Autodesk Inventor part; units mm, degrees
(part 2 of 3)
  spline S197 degree 2 poles (-17.3831, 5.9159) (-17.3831, 6.0168) (-17.518, 6.1517) (-17.6383, 6.1517) knots 0 0 0 1 2 2 2
  spline S198 degree 2 poles (-17.6383, 6.1517) (-17.7477, 6.1517) (-17.8875, 6.0314) (-17.8875, 5.928) knots 0 0 0 1 2 2 2
  spline S199 degree 2 poles (-17.8875, 5.928) (-17.8875, 5.8539) (-17.8158, 5.7506) (-17.7441, 5.7092) knots 0 0 0 1 2 2 2
  spline S200 degree 2 poles (-17.7441, 5.7092) (-17.7137, 5.6922) (-17.5848, 5.6327) (-17.5326, 5.6156) knots 0 0 0 1 2 2 2
  spline S201 degree 2 poles (-17.5326, 5.6156) (-17.4451, 5.6825) (-17.3831, 5.8247) (-17.3831, 5.9159) knots 0 0 0 1 2 2 2
  line L310 (-16.9748, 4.9432) -> (-16.6479, 4.9432)
  spline S202 degree 2 poles (-16.6479, 4.9432) (-16.9588, 5.2027) (-16.9588, 5.5777) knots 0 0 0 1 1 1
  spline S203 degree 2 poles (-16.9588, 5.5777) (-16.9588, 5.7812) (-16.7953, 6.1048) (-16.4958, 6.2923) (-16.2866, 6.2923) knots 0 0 0 1 2 3 3 3
  spline S204 degree 2 poles (-16.2866, 6.2923) (-16.0785, 6.2923) (-15.8018, 6.1208) (-15.6223, 5.7984) (-15.6223, 5.5777) knots 0 0 0 1 2 3 3 3
  spline S205 degree 2 poles (-15.6223, 5.5777) (-15.6223, 5.2027) (-15.9322, 4.9432) knots 0 0 0 1 1 1
  line L311 (-15.9322, 4.9432) -> (-15.6063, 4.9432)
  line L312 (-15.6063, 4.9432) -> (-15.6063, 4.766)
  line L313 (-15.6063, 4.766) -> (-16.1883, 4.766)
  line L314 (-16.1883, 4.766) -> (-16.1883, 4.9317)
  spline S206 degree 2 poles (-16.1883, 4.9317) (-15.8247, 5.1021) (-15.8247, 5.5468) knots 0 0 0 1 1 1
  spline S207 degree 2 poles (-15.8247, 5.5468) (-15.8247, 5.7972) (-16.0819, 6.1219) (-16.2877, 6.1219) knots 0 0 0 1 2 2 2
  spline S208 degree 2 poles (-16.2877, 6.1219) (-16.5004, 6.1219) (-16.7542, 5.7949) (-16.7542, 5.5571) knots 0 0 0 1 2 2 2
  spline S209 degree 2 poles (-16.7542, 5.5571) (-16.7542, 5.1055) (-16.3906, 4.9317) knots 0 0 0 1 1 1
  line L315 (-16.3906, 4.9317) -> (-16.3906, 4.766)
  line L316 (-16.3906, 4.766) -> (-16.9748, 4.766)
  line L317 (-16.9748, 4.766) -> (-16.9748, 4.9432)
  line L318 (-14.3756, 5.0335) -> (-14.3756, 5.4451)
  line L319 (-14.3756, 5.4451) -> (-14.7837, 5.4451)
  line L320 (-14.7837, 5.4451) -> (-14.7837, 5.6154)
  line L321 (-14.7837, 5.6154) -> (-14.3756, 5.6154)
  line L322 (-14.3756, 5.6154) -> (-14.3756, 6.0236)
  line L323 (-14.3756, 6.0236) -> (-14.2018, 6.0236)
  line L324 (-14.2018, 6.0236) -> (-14.2018, 5.6154)
  line L325 (-14.2018, 5.6154) -> (-13.7936, 5.6154)
  line L326 (-13.7936, 5.6154) -> (-13.7936, 5.4451)
  line L327 (-13.7936, 5.4451) -> (-14.2018, 5.4451)
  line L328 (-14.2018, 5.4451) -> (-14.2018, 5.0335)
  line L329 (-14.2018, 5.0335) -> (-14.3756, 5.0335)
  line L330 (-13.7936, 4.766) -> (-14.7837, 4.766)
  line L331 (-14.7837, 4.766) -> (-14.7837, 4.9375)
  line L332 (-14.7837, 4.9375) -> (-13.7936, 4.9375)
  line L333 (-13.7936, 4.9375) -> (-13.7936, 4.766)
  line L334 (-12.1726, 4.766) -> (-12.9044, 4.766)
  line L335 (-12.9044, 4.766) -> (-12.9044, 4.9191)
  line L336 (-12.9044, 4.9191) -> (-12.6321, 4.9191)
  line L337 (-12.6321, 4.9191) -> (-12.6321, 5.9244)
  line L338 (-12.6321, 5.9244) -> (-12.9044, 5.9244)
  line L339 (-12.9044, 5.9244) -> (-12.9044, 6.0618)
  spline S210 degree 2 poles (-12.9044, 6.0618) (-12.75, 6.0618) (-12.6041, 6.1493) (-12.5944, 6.2708) knots 0 0 0 1 2 2 2
  line L340 (-12.5944, 6.2708) -> (-12.4388, 6.2708)
  line L341 (-12.4388, 6.2708) -> (-12.4388, 4.9191)
  line L342 (-12.4388, 4.9191) -> (-12.1726, 4.9191)
  line L343 (-12.1726, 4.9191) -> (-12.1726, 4.766)
  spline S211 degree 2 poles (-10.9631, 5.516) (-10.9631, 5.1124) (-11.1977, 4.7344) (-11.442, 4.7344) knots 0 0 0 1 2 2 2
  spline S212 degree 2 poles (-11.442, 4.7344) (-11.69, 4.7344) (-11.9222, 5.1197) (-11.9222, 5.5147) knots 0 0 0 1 2 2 2
  spline S213 degree 2 poles (-11.9222, 5.5147) (-11.9222, 5.9207) (-11.6876, 6.2964) (-11.442, 6.2964) knots 0 0 0 1 2 2 2
  spline S214 degree 2 poles (-11.442, 6.2964) (-11.1953, 6.2964) (-10.9631, 5.9074) (-10.9631, 5.516) knots 0 0 0 1 2 2 2
  spline S215 degree 2 poles (-11.2208, 5.0589) (-11.1916, 5.1331) (-11.1673, 5.3616) (-11.1673, 5.516) knots 0 0 0 1 2 2 2
  spline S216 degree 2 poles (-11.1673, 5.516) (-11.1673, 5.6703) (-11.1916, 5.8976) (-11.222, 5.9742) knots 0 0 0 1 2 2 2
  spline S217 degree 2 poles (-11.222, 5.9742) (-11.2524, 6.0508) (-11.3582, 6.1298) (-11.442, 6.1298) knots 0 0 0 1 2 2 2
  spline S218 degree 2 poles (-11.442, 6.1298) (-11.5259, 6.1298) (-11.6341, 6.0508) (-11.6657, 5.9718) knots 0 0 0 1 2 2 2
  spline S219 degree 2 poles (-11.6657, 5.9718) (-11.6961, 5.8952) (-11.718, 5.6618) (-11.718, 5.5147) knots 0 0 0 1 2 2 2
  spline S220 degree 2 poles (-11.718, 5.5147) (-11.718, 5.3567) (-11.6985, 5.1452) (-11.6669, 5.0626) knots 0 0 0 1 2 2 2
  spline S221 degree 2 poles (-11.6669, 5.0626) (-11.6377, 4.9848) (-11.5296, 4.9009) (-11.442, 4.9009) knots 0 0 0 1 2 2 2
  spline S222 degree 2 poles (-11.442, 4.9009) (-11.3594, 4.9009) (-11.2512, 4.9799) (-11.2208, 5.0589) knots 0 0 0 1 2 2 2
  spline S223 degree 2 poles (-8.9696, 5.1817) (-8.9696, 4.9556) (-9.1519, 4.7368) (-9.3245, 4.7368) knots 0 0 0 1 2 2 2
  spline S224 degree 2 poles (-9.3245, 4.7368) (-9.4996, 4.7368) (-9.6795, 4.958) (-9.6795, 5.1817) knots 0 0 0 1 2 2 2
  spline S225 degree 2 poles (-9.6795, 5.1817) (-9.6795, 5.4066) (-9.4959, 5.6266) (-9.3245, 5.6266) knots 0 0 0 1 2 2 2
  spline S226 degree 2 poles (-9.3245, 5.6266) (-9.1483, 5.6266) (-8.9696, 5.4053) (-8.9696, 5.1817) knots 0 0 0 1 2 2 2
  spline S227 degree 2 poles (-10.0672, 5.849) (-10.0672, 5.6229) (-10.2496, 5.4041) (-10.4222, 5.4041) knots 0 0 0 1 2 2 2
  spline S228 degree 2 poles (-10.4222, 5.4041) (-10.5972, 5.4041) (-10.7771, 5.6254) (-10.7771, 5.849) knots 0 0 0 1 2 2 2
  spline S229 degree 2 poles (-10.7771, 5.849) (-10.7771, 6.0739) (-10.5936, 6.2939) (-10.4222, 6.2939) knots 0 0 0 1 2 2 2
  spline S230 degree 2 poles (-10.4222, 6.2939) (-10.2459, 6.2939) (-10.0672, 6.0727) (-10.0672, 5.849) knots 0 0 0 1 2 2 2
  line L344 (-9.3963, 6.266) -> (-10.1815, 4.766)
  line L345 (-10.1815, 4.766) -> (-10.348, 4.766)
  line L346 (-10.348, 4.766) -> (-9.5628, 6.266)
  line L347 (-9.5628, 6.266) -> (-9.3963, 6.266)
  spline S231 degree 2 poles (-9.1483, 5.1817) (-9.1483, 5.3361) (-9.22, 5.4929) (-9.3233, 5.4929) knots 0 0 0 1 2 2 2
  spline S232 degree 2 poles (-9.3233, 5.4929) (-9.4266, 5.4929) (-9.4996, 5.3336) (-9.4996, 5.1817) knots 0 0 0 1 2 2 2
  spline S233 degree 2 poles (-9.4996, 5.1817) (-9.4996, 5.0297) (-9.4315, 4.8705) (-9.3233, 4.8705) knots 0 0 0 1 2 2 2
  spline S234 degree 2 poles (-9.3233, 4.8705) (-9.22, 4.8705) (-9.1483, 5.0297) (-9.1483, 5.1817) knots 0 0 0 1 2 2 2
  spline S235 degree 2 poles (-10.2459, 5.849) (-10.2459, 6.0034) (-10.3176, 6.1602) (-10.421, 6.1602) knots 0 0 0 1 2 2 2
  spline S236 degree 2 poles (-10.421, 6.1602) (-10.5243, 6.1602) (-10.5972, 6.001) (-10.5972, 5.849) knots 0 0 0 1 2 2 2
  spline S237 degree 2 poles (-10.5972, 5.849) (-10.5972, 5.6971) (-10.5292, 5.5378) (-10.421, 5.5378) knots 0 0 0 1 2 2 2
  spline S238 degree 2 poles (-10.421, 5.5378) (-10.3176, 5.5378) (-10.2459, 5.6971) (-10.2459, 5.849) knots 0 0 0 1 2 2 2
  spline S239 degree 2 poles (7.5525, 5.8211) (7.5525, 5.7238) (7.4832, 5.5488) (7.4213, 5.488) knots 0 0 0 1 2 2 2
  spline S240 degree 2 poles (7.4213, 5.488) (7.3435, 5.4114) (7.1332, 5.3324) (6.9727, 5.3324) knots 0 0 0 1 2 2 2
  line L348 (6.9727, 5.3324) -> (6.8038, 5.3324)
  line L349 (6.8038, 5.3324) -> (6.8038, 4.7733)
  line L350 (6.8038, 4.7733) -> (6.6044, 4.7733)
  line L351 (6.6044, 4.7733) -> (6.6044, 6.2733)
  line L352 (6.6044, 6.2733) -> (6.9812, 6.2733)
  spline S241 degree 2 poles (6.9812, 6.2733) (7.1149, 6.2733) (7.3021, 6.2295) (7.3738, 6.1797) knots 0 0 0 1 2 2 2
  spline S242 degree 2 poles (7.3738, 6.1797) (7.4577, 6.1225) (7.5525, 5.9463) (7.5525, 5.8211) knots 0 0 0 1 2 2 2
  spline S243 degree 2 poles (7.3447, 5.815) (7.3447, 5.8928) (7.2912, 6.0071) (7.2365, 6.0435) knots 0 0 0 1 2 2 2
  spline S244 degree 2 poles (7.2365, 6.0435) (7.1891, 6.0751) (7.0627, 6.1006) (6.9691, 6.1006) knots 0 0 0 1 2 2 2
  line L353 (6.9691, 6.1006) -> (6.8038, 6.1006)
  line L354 (6.8038, 6.1006) -> (6.8038, 5.5026)
  line L355 (6.8038, 5.5026) -> (6.9399, 5.5026)
  spline S245 degree 2 poles (6.9399, 5.5026) (7.0614, 5.5026) (7.211, 5.5415) (7.2596, 5.5925) knots 0 0 0 1 2 2 2
  spline S246 degree 2 poles (7.2596, 5.5925) (7.3046, 5.6375) (7.3447, 5.7433) (7.3447, 5.815) knots 0 0 0 1 2 2 2
  spline S247 degree 2 poles (8.2661, 4.7417) (8.1336, 4.7417) (7.9367, 4.8109) (7.8674, 4.8802) knots 0 0 0 1 2 2 2
  spline S248 degree 2 poles (7.8674, 4.8802) (7.7884, 4.958) (7.7239, 5.1768) (7.7239, 5.3373) knots 0 0 0 1 2 2 2
  line L356 (7.7239, 5.3373) -> (7.7239, 6.2733)
  line L357 (7.7239, 6.2733) -> (7.9233, 6.2733)
  line L358 (7.9233, 6.2733) -> (7.9233, 5.3373)
  spline S249 degree 2 poles (7.9233, 5.3373) (7.9233, 5.2327) (7.95, 5.0917) (7.9877, 5.0346) knots 0 0 0 1 2 2 2
  spline S250 degree 2 poles (7.9877, 5.0346) (8.0278, 4.9738) (8.1664, 4.9118) (8.2661, 4.9118) knots 0 0 0 1 2 2 2
  spline S251 degree 2 poles (8.2661, 4.9118) (8.3597, 4.9118) (8.5055, 4.9738) (8.5456, 5.0346) knots 0 0 0 1 2 2 2
  spline S252 degree 2 poles (8.5456, 5.0346) (8.5833, 5.0917) (8.6101, 5.2315) (8.6101, 5.3324) knots 0 0 0 1 2 2 2
  line L359 (8.6101, 5.3324) -> (8.6101, 6.2733)
  line L360 (8.6101, 6.2733) -> (8.8094, 6.2733)
  line L361 (8.8094, 6.2733) -> (8.8094, 5.3373)
  spline S253 degree 2 poles (8.8094, 5.3373) (8.8094, 5.1805) (8.7462, 4.9568) (8.666, 4.8802) knots 0 0 0 1 2 2 2
  spline S254 degree 2 poles (8.666, 4.8802) (8.5943, 4.8097) (8.4046, 4.7417) (8.2661, 4.7417) knots 0 0 0 1 2 2 2
  spline S255 degree 2 poles (9.5132, 4.7465) (9.3503, 4.7465) (9.1218, 4.8146) (9.0209, 4.8632) knots 0 0 0 1 2 2 2
  line L362 (9.0209, 4.8632) -> (9.0209, 5.1136)
  line L363 (9.0209, 5.1136) -> (9.0355, 5.1136)
  spline S256 degree 2 poles (9.0355, 5.1136) (9.134, 5.0212) (9.3832, 4.9191) (9.4986, 4.9191) knots 0 0 0 1 2 2 2
  spline S257 degree 2 poles (9.4986, 4.9191) (9.664, 4.9191) (9.8329, 5.0565) (9.8329, 5.1695) knots 0 0 0 1 2 2 2
  spline S258 degree 2 poles (9.8329, 5.1695) (9.8329, 5.2595) (9.7442, 5.3713) (9.6482, 5.3993) knots 0 0 0 1 2 2 2
  spline S259 degree 2 poles (9.6482, 5.3993) (9.5789, 5.4187) (9.4634, 5.4455) (9.3771, 5.4673) knots 0 0 0 1 2 2 2
  spline S260 degree 2 poles (9.3771, 5.4673) (9.2993, 5.488) (9.1765, 5.55) (9.1291, 5.5998) knots 0 0 0 1 2 2 2
  spline S261 degree 2 poles (9.1291, 5.5998) (9.0829, 5.6497) (9.0319, 5.7834) (9.0319, 5.8709) knots 0 0 0 1 2 2 2
  spline S262 degree 2 poles (9.0319, 5.8709) (9.0319, 6.0532) (9.3163, 6.3) (9.5363, 6.3) knots 0 0 0 1 2 2 2
  spline S263 degree 2 poles (9.5363, 6.3) (9.6627, 6.3) (9.8864, 6.2502) (9.9824, 6.2028) knots 0 0 0 1 2 2 2
  line L364 (9.9824, 6.2028) -> (9.9824, 5.9645)
  line L365 (9.9824, 5.9645) -> (9.9679, 5.9645)
  spline S264 degree 2 poles (9.9679, 5.9645) (9.8961, 6.0301) (9.6725, 6.1274) (9.5497, 6.1274) knots 0 0 0 1 2 2 2
  spline S265 degree 2 poles (9.5497, 6.1274) (9.4111, 6.1274) (9.2397, 5.9973) (9.2397, 5.8916) knots 0 0 0 1 2 2 2
  spline S266 degree 2 poles (9.2397, 5.8916) (9.2397, 5.7968) (9.3406, 5.6837) (9.4354, 5.6582) knots 0 0 0 1 2 2 2
  spline S267 degree 2 poles (9.4354, 5.6582) (9.4986, 5.6412) (9.6822, 5.5974) (9.743, 5.5792) knots 0 0 0 1 2 2 2
  spline S268 degree 2 poles (9.743, 5.5792) (9.8973, 5.5318) (10.0408, 5.3409) (10.0408, 5.2011) knots 0 0 0 1 2 2 2
  spline S269 degree 2 poles (10.0408, 5.2011) (10.0408, 5.1124) (9.9691, 4.9422) (9.9046, 4.8827) knots 0 0 0 1 2 2 2
  spline S270 degree 2 poles (9.9046, 4.8827) (9.8329, 4.817) (9.6506, 4.7465) (9.5132, 4.7465) knots 0 0 0 1 2 2 2
  line L366 (11.3329, 4.7733) -> (11.1336, 4.7733)
  line L367 (11.1336, 4.7733) -> (11.1336, 5.5075)
  line L368 (11.1336, 5.5075) -> (10.4431, 5.5075)
  line L369 (10.4431, 5.5075) -> (10.4431, 4.7733)
  line L370 (10.4431, 4.7733) -> (10.2438, 4.7733)
  line L371 (10.2438, 4.7733) -> (10.2438, 6.2733)
  line L372 (10.2438, 6.2733) -> (10.4431, 6.2733)
  line L373 (10.4431, 6.2733) -> (10.4431, 5.6849)
  line L374 (10.4431, 5.6849) -> (11.1336, 5.6849)
  line L375 (11.1336, 5.6849) -> (11.1336, 6.2733)
  line L376 (11.1336, 6.2733) -> (11.3329, 6.2733)
  line L377 (11.3329, 6.2733) -> (11.3329, 4.7733)
  line L378 (-21.1508, 14.6571) -> (-22.3097, 14.6571)
  line L379 (-22.3097, 14.6571) -> (-22.3097, 16.6571)
  line L380 (-22.3097, 16.6571) -> (-22.0439, 16.6571)
  line L381 (-22.0439, 16.6571) -> (-22.0439, 14.8937)
  line L382 (-22.0439, 14.8937) -> (-21.1508, 14.8937)
  line L383 (-21.1508, 14.8937) -> (-21.1508, 14.6571)
  spline S271 degree 2 poles (-19.5268, 16.4285) (-19.4134, 16.2956) (-19.287, 15.9067) (-19.287, 15.6571) knots 0 0 0 1 2 2 2
  spline S272 degree 2 poles (-19.287, 15.6571) (-19.287, 15.414) (-19.4101, 15.0201) (-19.5268, 14.8872) knots 0 0 0 1 2 2 2
  spline S273 degree 2 poles (-19.5268, 14.8872) (-19.65, 14.7478) (-19.9758, 14.6149) (-20.1719, 14.6149) knots 0 0 0 1 2 2 2
  spline S274 degree 2 poles (-20.1719, 14.6149) (-20.3745, 14.6149) (-20.6986, 14.7527) (-20.8169, 14.8872) knots 0 0 0 1 2 2 2
  spline S275 degree 2 poles (-20.8169, 14.8872) (-20.932, 15.0201) (-21.0552, 15.4107) (-21.0552, 15.6571) knots 0 0 0 1 2 2 2
  spline S276 degree 2 poles (-21.0552, 15.6571) (-21.0552, 15.9083) (-20.9304, 16.2908) (-20.8153, 16.4285) knots 0 0 0 1 2 2 2
  spline S277 degree 2 poles (-20.8153, 16.4285) (-20.6986, 16.5614) (-20.3729, 16.6992) (-20.1719, 16.6992) knots 0 0 0 1 2 2 2
  spline S278 degree 2 poles (-20.1719, 16.6992) (-19.9677, 16.6992) (-19.6403, 16.5566) (-19.5268, 16.4285) knots 0 0 0 1 2 2 2
  spline S279 degree 2 poles (-19.5641, 15.6571) (-19.5641, 15.8548) (-19.65, 16.1611) (-19.7278, 16.2616) knots 0 0 0 1 2 2 2
  spline S280 degree 2 poles (-19.7278, 16.2616) (-19.8072, 16.3653) (-20.0309, 16.4691) (-20.1703, 16.4691) knots 0 0 0 1 2 2 2
  spline S281 degree 2 poles (-20.1703, 16.4691) (-20.3145, 16.4691) (-20.5317, 16.3686) (-20.6144, 16.2616) knots 0 0 0 1 2 2 2
  spline S282 degree 2 poles (-20.6144, 16.2616) (-20.6938, 16.1595) (-20.778, 15.8516) (-20.778, 15.6571) knots 0 0 0 1 2 2 2
  spline S283 degree 2 poles (-20.778, 15.6571) (-20.778, 15.2632) (-20.4474, 14.8451) (-20.1703, 14.8451) knots 0 0 0 1 2 2 2
  spline S284 degree 2 poles (-20.1703, 14.8451) (-19.8931, 14.8451) (-19.5641, 15.2632) (-19.5641, 15.6571) knots 0 0 0 1 2 2 2
  line L384 (-19.2108, 14.6571) -> (-18.5366, 16.6571)
  line L385 (-18.5366, 16.6571) -> (-18.2092, 16.6571)
  line L386 (-18.2092, 16.6571) -> (-17.5349, 14.6571)
  line L387 (-17.5349, 14.6571) -> (-17.8153, 14.6571)
  line L388 (-17.8153, 14.6571) -> (-17.9968, 15.2162)
  line L389 (-17.9968, 15.2162) -> (-18.7602, 15.2162)
  line L390 (-18.7602, 15.2162) -> (-18.9417, 14.6571)
  line L391 (-18.9417, 14.6571) -> (-19.2108, 14.6571)
  line L392 (-18.0698, 15.4431) -> (-18.3793, 16.3848)
  line L393 (-18.3793, 16.3848) -> (-18.6873, 15.4431)
  line L394 (-18.6873, 15.4431) -> (-18.0698, 15.4431)
  spline S285 degree 2 poles (-15.7683, 15.6554) (-15.7683, 15.3815) (-15.9904, 14.9407) (-16.1768, 14.8175) knots 0 0 0 1 2 2 2
  spline S286 degree 2 poles (-16.1768, 14.8175) (-16.3291, 14.7219) (-16.6419, 14.6571) (-16.885, 14.6571) knots 0 0 0 1 2 2 2
  line L395 (-16.885, 14.6571) -> (-17.3453, 14.6571)
  line L396 (-17.3453, 14.6571) -> (-17.3453, 16.6571)
  line L397 (-17.3453, 16.6571) -> (-16.8899, 16.6571)
  spline S287 degree 2 poles (-16.8899, 16.6571) (-16.6079, 16.6571) (-16.287, 16.5728) (-16.1735, 16.4982) knots 0 0 0 1 2 2 2
  spline S288 degree 2 poles (-16.1735, 16.4982) (-15.9806, 16.3702) (-15.7683, 15.9472) (-15.7683, 15.6554) knots 0 0 0 1 2 2 2
  spline S289 degree 2 poles (-16.0455, 15.6587) (-16.0455, 15.8888) (-16.1978, 16.2146) (-16.3486, 16.307) knots 0 0 0 1 2 2 2
  spline S290 degree 2 poles (-16.3486, 16.307) (-16.4555, 16.3702) (-16.697, 16.4269) (-16.8769, 16.4269) knots 0 0 0 1 2 2 2
  line L398 (-16.8769, 16.4269) -> (-17.0795, 16.4269)
  line L399 (-17.0795, 16.4269) -> (-17.0795, 14.8872)
  line L400 (-17.0795, 14.8872) -> (-16.8769, 14.8872)
  spline S291 degree 2 poles (-16.8769, 14.8872) (-16.7003, 14.8872) (-16.4328, 14.9439) (-16.3242, 15.0201) knots 0 0 0 1 2 2 2
  spline S292 degree 2 poles (-16.3242, 15.0201) (-16.1849, 15.1141) (-16.0455, 15.4253) (-16.0455, 15.6587) knots 0 0 0 1 2 2 2
  spline S293 degree 2 poles (-13.8396, 14.6214) (-14.0341, 14.6214) (-14.3631, 14.7527) (-14.4831, 14.884) knots 0 0 0 1 2 2 2
  spline S294 degree 2 poles (-14.4831, 14.884) (-14.603, 15.0136) (-14.7343, 15.4026) (-14.7343, 15.6554) knots 0 0 0 1 2 2 2
  spline S295 degree 2 poles (-14.7343, 15.6554) (-14.7343, 15.9067) (-14.6063, 16.2794) (-14.4847, 16.4172) knots 0 0 0 1 2 2 2
  spline S296 degree 2 poles (-14.4847, 16.4172) (-14.3648, 16.5517) (-14.0374, 16.6927) (-13.8348, 16.6927) knots 0 0 0 1 2 2 2
  spline S297 degree 2 poles (-13.8348, 16.6927) (-13.7343, 16.6927) (-13.5576, 16.6636) (-13.4831, 16.6409) knots 0 0 0 1 2 2 2
  spline S298 degree 2 poles (-13.4831, 16.6409) (-13.4182, 16.6198) (-13.2837, 16.5598) (-13.2173, 16.5242) knots 0 0 0 1 2 2 2
  line L401 (-13.2173, 16.5242) -> (-13.2173, 16.2033)
  line L402 (-13.2173, 16.2033) -> (-13.2383, 16.2033)
  spline S299 degree 2 poles (-13.2383, 16.2033) (-13.274, 16.2357) (-13.3842, 16.3264) (-13.4636, 16.3702) knots 0 0 0 1 2 2 2
  spline S300 degree 2 poles (-13.4636, 16.3702) (-13.5398, 16.4123) (-13.7197, 16.4658) (-13.8364, 16.4658) knots 0 0 0 1 2 2 2
  spline S301 degree 2 poles (-13.8364, 16.4658) (-13.9644, 16.4658) (-14.193, 16.3605) (-14.2789, 16.26) knots 0 0 0 1 2 2 2
  spline S302 degree 2 poles (-14.2789, 16.26) (-14.3631, 16.1579) (-14.4571, 15.8483) (-14.4571, 15.6554) knots 0 0 0 1 2 2 2
  spline S303 degree 2 poles (-14.4571, 15.6554) (-14.4571, 15.4496) (-14.3583, 15.153) (-14.2724, 15.0509) knots 0 0 0 1 2 2 2
  spline S304 degree 2 poles (-14.2724, 15.0509) (-14.1881, 14.952) (-13.9628, 14.8516) (-13.8364, 14.8516) knots 0 0 0 1 2 2 2
  spline S305 degree 2 poles (-13.8364, 14.8516) (-13.7213, 14.8516) (-13.5252, 14.9083) (-13.449, 14.9504) knots 0 0 0 1 2 2 2
  spline S306 degree 2 poles (-13.449, 14.9504) (-13.3761, 14.9926) (-13.2675, 15.0801) (-13.2367, 15.1109) knots 0 0 0 1 2 2 2
  line L403 (-13.2367, 15.1109) -> (-13.2173, 15.1109)
  line L404 (-13.2173, 15.1109) -> (-13.2173, 14.7932)
  spline S307 degree 2 poles (-13.2173, 14.7932) (-13.2837, 14.7624) (-13.4004, 14.7057) (-13.4831, 14.6798) knots 0 0 0 1 2 2 2
  spline S308 degree 2 poles (-13.4831, 14.6798) (-13.5706, 14.6506) (-13.7197, 14.6214) (-13.8396, 14.6214) knots 0 0 0 1 2 2 2
  line L405 (-11.5171, 14.6571) -> (-11.7829, 14.6571)
  line L406 (-11.7829, 14.6571) -> (-11.7829, 15.636)
  line L407 (-11.7829, 15.636) -> (-12.7035, 15.636)
  line L408 (-12.7035, 15.636) -> (-12.7035, 14.6571)
  line L409 (-12.7035, 14.6571) -> (-12.9693, 14.6571)
  line L410 (-12.9693, 14.6571) -> (-12.9693, 16.6571)
  line L411 (-12.9693, 16.6571) -> (-12.7035, 16.6571)
  line L412 (-12.7035, 16.6571) -> (-12.7035, 15.8726)
  line L413 (-12.7035, 15.8726) -> (-11.7829, 15.8726)
  line L414 (-11.7829, 15.8726) -> (-11.7829, 16.6571)
  line L415 (-11.7829, 16.6571) -> (-11.5171, 16.6571)
  line L416 (-11.5171, 16.6571) -> (-11.5171, 14.6571)
  line L417 (-11.1119, 14.6571) -> (-11.1119, 16.6571)
  line L418 (-11.1119, 16.6571) -> (-9.8607, 16.6571)
  line L419 (-9.8607, 16.6571) -> (-9.8607, 16.4204)
  line L420 (-9.8607, 16.4204) -> (-10.8461, 16.4204)
  line L421 (-10.8461, 16.4204) -> (-10.8461, 15.8726)
  line L422 (-10.8461, 15.8726) -> (-9.9272, 15.8726)
  line L423 (-9.9272, 15.8726) -> (-9.9272, 15.636)
  line L424 (-9.9272, 15.636) -> (-10.8461, 15.636)
  line L425 (-10.8461, 15.636) -> (-10.8461, 14.8937)
  line L426 (-10.8461, 14.8937) -> (-9.8607, 14.8937)
  line L427 (-9.8607, 14.8937) -> (-9.8607, 14.6571)
  line L428 (-9.8607, 14.6571) -> (-11.1119, 14.6571)
  spline S309 degree 2 poles (-8.7878, 14.6214) (-8.9823, 14.6214) (-9.3113, 14.7527) (-9.4312, 14.884) knots 0 0 0 1 2 2 2
  spline S310 degree 2 poles (-9.4312, 14.884) (-9.5511, 15.0136) (-9.6824, 15.4026) (-9.6824, 15.6554) knots 0 0 0 1 2 2 2
  spline S311 degree 2 poles (-9.6824, 15.6554) (-9.6824, 15.9067) (-9.5544, 16.2794) (-9.4328, 16.4172) knots 0 0 0 1 2 2 2
  spline S312 degree 2 poles (-9.4328, 16.4172) (-9.3129, 16.5517) (-8.9855, 16.6927) (-8.7829, 16.6927) knots 0 0 0 1 2 2 2
  spline S313 degree 2 poles (-8.7829, 16.6927) (-8.6824, 16.6927) (-8.5058, 16.6636) (-8.4312, 16.6409) knots 0 0 0 1 2 2 2
  spline S314 degree 2 poles (-8.4312, 16.6409) (-8.3664, 16.6198) (-8.2319, 16.5598) (-8.1654, 16.5242) knots 0 0 0 1 2 2 2
  line L429 (-8.1654, 16.5242) -> (-8.1654, 16.2033)
  line L430 (-8.1654, 16.2033) -> (-8.1865, 16.2033)
  spline S315 degree 2 poles (-8.1865, 16.2033) (-8.2221, 16.2357) (-8.3323, 16.3264) (-8.4118, 16.3702) knots 0 0 0 1 2 2 2
  spline S316 degree 2 poles (-8.4118, 16.3702) (-8.4879, 16.4123) (-8.6678, 16.4658) (-8.7845, 16.4658) knots 0 0 0 1 2 2 2
  spline S317 degree 2 poles (-8.7845, 16.4658) (-8.9126, 16.4658) (-9.1411, 16.3605) (-9.227, 16.26) knots 0 0 0 1 2 2 2
  spline S318 degree 2 poles (-9.227, 16.26) (-9.3113, 16.1579) (-9.4053, 15.8483) (-9.4053, 15.6554) knots 0 0 0 1 2 2 2
  spline S319 degree 2 poles (-9.4053, 15.6554) (-9.4053, 15.4496) (-9.3064, 15.153) (-9.2205, 15.0509) knots 0 0 0 1 2 2 2
  spline S320 degree 2 poles (-9.2205, 15.0509) (-9.1362, 14.952) (-8.911, 14.8516) (-8.7845, 14.8516) knots 0 0 0 1 2 2 2
  spline S321 degree 2 poles (-8.7845, 14.8516) (-8.6695, 14.8516) (-8.4733, 14.9083) (-8.3972, 14.9504) knots 0 0 0 1 2 2 2
  spline S322 degree 2 poles (-8.3972, 14.9504) (-8.3242, 14.9926) (-8.2157, 15.0801) (-8.1849, 15.1109) knots 0 0 0 1 2 2 2
  line L431 (-8.1849, 15.1109) -> (-8.1654, 15.1109)
  line L432 (-8.1654, 15.1109) -> (-8.1654, 14.7932)
  spline S323 degree 2 poles (-8.1654, 14.7932) (-8.2319, 14.7624) (-8.3486, 14.7057) (-8.4312, 14.6798) knots 0 0 0 1 2 2 2
  spline S324 degree 2 poles (-8.4312, 14.6798) (-8.5187, 14.6506) (-8.6678, 14.6214) (-8.7878, 14.6214) knots 0 0 0 1 2 2 2
  line L433 (-6.4588, 14.6571) -> (-6.804, 14.6571)
  line L434 (-6.804, 14.6571) -> (-7.5349, 15.5874)
  line L435 (-7.5349, 15.5874) -> (-7.6516, 15.4561)
  line L436 (-7.6516, 15.4561) -> (-7.6516, 14.6571)
  line L437 (-7.6516, 14.6571) -> (-7.9174, 14.6571)
  line L438 (-7.9174, 14.6571) -> (-7.9174, 16.6571)
  line L439 (-7.9174, 16.6571) -> (-7.6516, 16.6571)
  line L440 (-7.6516, 16.6571) -> (-7.6516, 15.7381)
  line L441 (-7.6516, 15.7381) -> (-6.8315, 16.6571)
  line L442 (-6.8315, 16.6571) -> (-6.5074, 16.6571)
  line L443 (-6.5074, 16.6571) -> (-7.3356, 15.764)
  line L444 (-7.3356, 15.764) -> (-6.4588, 14.6571)
  line L445 (8.5156, 14.6636) -> (8.1704, 14.6636)
  line L446 (8.1704, 14.6636) -> (7.5383, 15.4593)
  line L447 (7.5383, 15.4593) -> (7.2336, 15.4593)
  line L448 (7.2336, 15.4593) -> (7.2336, 14.6636)
  line L449 (7.2336, 14.6636) -> (6.9678, 14.6636)
  line L450 (6.9678, 14.6636) -> (6.9678, 16.6636)
  line L451 (6.9678, 16.6636) -> (7.4832, 16.6636)
  spline S325 degree 2 poles (7.4832, 16.6636) (7.655, 16.6636) (7.8868, 16.6263) (7.9921, 16.5582) knots 0 0 0 1 2 2 2
  spline S326 degree 2 poles (7.9921, 16.5582) (8.0975, 16.4901) (8.219, 16.2778) (8.219, 16.1206) knots 0 0 0 1 2 2 2
  spline S327 degree 2 poles (8.219, 16.1206) (8.219, 15.9018) (7.9954, 15.6052) (7.8041, 15.5339) knots 0 0 0 1 2 2 2
  line L452 (7.8041, 15.5339) -> (8.5156, 14.6636)
  spline S328 degree 2 poles (7.9419, 16.0995) (7.9419, 16.1871) (7.8803, 16.3216) (7.8155, 16.3653) knots 0 0 0 1 2 2 2
  spline S329 degree 2 poles (7.8155, 16.3653) (7.7587, 16.4026) (7.608, 16.4334) (7.4978, 16.4334) knots 0 0 0 1 2 2 2
  line L453 (7.4978, 16.4334) -> (7.2336, 16.4334)
  line L454 (7.2336, 16.4334) -> (7.2336, 15.6814)
  line L455 (7.2336, 15.6814) -> (7.467, 15.6814)
  spline S330 degree 2 poles (7.467, 15.6814) (7.5821, 15.6814) (7.7652, 15.7219) (7.8284, 15.7851) knots 0 0 0 1 2 2 2
  spline S331 degree 2 poles (7.8284, 15.7851) (7.8868, 15.8402) (7.9419, 15.9958) (7.9419, 16.0995) knots 0 0 0 1 2 2 2
  line L456 (8.6745, 14.6636) -> (8.6745, 16.6636)
  line L457 (8.6745, 16.6636) -> (9.9257, 16.6636)
  line L458 (9.9257, 16.6636) -> (9.9257, 16.4269)
  line L459 (9.9257, 16.4269) -> (8.9403, 16.4269)
  line L460 (8.9403, 16.4269) -> (8.9403, 15.8791)
  line L461 (8.9403, 15.8791) -> (9.8592, 15.8791)
  line L462 (9.8592, 15.8791) -> (9.8592, 15.6425)
  line L463 (9.8592, 15.6425) -> (8.9403, 15.6425)
  line L464 (8.9403, 15.6425) -> (8.9403, 14.9002)
  line L465 (8.9403, 14.9002) -> (9.9257, 14.9002)
  line L466 (9.9257, 14.9002) -> (9.9257, 14.6636)
  line L467 (9.9257, 14.6636) -> (8.6745, 14.6636)
  line L468 (11.3762, 14.6636) -> (10.2174, 14.6636)
  line L469 (10.2174, 14.6636) -> (10.2174, 16.6636)
  line L470 (10.2174, 16.6636) -> (10.4832, 16.6636)
  line L471 (10.4832, 16.6636) -> (10.4832, 14.9002)
  line L472 (10.4832, 14.9002) -> (11.3762, 14.9002)
  line L473 (11.3762, 14.9002) -> (11.3762, 14.6636)
  line L474 (11.3698, 14.6636) -> (12.044, 16.6636)
  line L475 (12.044, 16.6636) -> (12.3714, 16.6636)
  line L476 (12.3714, 16.6636) -> (13.0456, 14.6636)
  line L477 (13.0456, 14.6636) -> (12.7652, 14.6636)
  line L478 (12.7652, 14.6636) -> (12.5837, 15.2227)
  line L479 (12.5837, 15.2227) -> (11.8203, 15.2227)
  line L480 (11.8203, 15.2227) -> (11.6388, 14.6636)
  line L481 (11.6388, 14.6636) -> (11.3698, 14.6636)
  line L482 (12.5108, 15.4496) -> (12.2012, 16.3913)
  line L483 (12.2012, 16.3913) -> (11.8933, 15.4496)
  line L484 (11.8933, 15.4496) -> (12.5108, 15.4496)
  line L485 (14.6356, 16.6636) -> (13.9597, 15.5485)
  line L486 (13.9597, 15.5485) -> (13.9597, 14.6636)
  line L487 (13.9597, 14.6636) -> (13.6939, 14.6636)
  line L488 (13.6939, 14.6636) -> (13.6939, 15.5209)
  line L489 (13.6939, 15.5209) -> (13.0181, 16.6636)
  line L490 (13.0181, 16.6636) -> (13.313, 16.6636)
  line L491 (13.313, 16.6636) -> (13.8284, 15.7835)
  line L492 (13.8284, 15.7835) -> (14.3536, 16.6636)
  line L493 (14.3536, 16.6636) -> (14.6356, 16.6636)
  spline S332 degree 2 poles (16.4605, 14.6279) (16.266, 14.6279) (15.937, 14.7592) (15.8171, 14.8905) knots 0 0 0 1 2 2 2
  spline S333 degree 2 poles (15.8171, 14.8905) (15.6972, 15.0201) (15.5659, 15.4091) (15.5659, 15.6619) knots 0 0 0 1 2 2 2
  spline S334 degree 2 poles (15.5659, 15.6619) (15.5659, 15.9131) (15.6939, 16.2859) (15.8155, 16.4237) knots 0 0 0 1 2 2 2
  spline S335 degree 2 poles (15.8155, 16.4237) (15.9354, 16.5582) (16.2628, 16.6992) (16.4654, 16.6992) knots 0 0 0 1 2 2 2
  spline S336 degree 2 poles (16.4654, 16.6992) (16.5659, 16.6992) (16.7425, 16.67) (16.8171, 16.6473) knots 0 0 0 1 2 2 2
  spline S337 degree 2 poles (16.8171, 16.6473) (16.8819, 16.6263) (17.0164, 16.5663) (17.0829, 16.5307) knots 0 0 0 1 2 2 2
  line L494 (17.0829, 16.5307) -> (17.0829, 16.2097)
  line L495 (17.0829, 16.2097) -> (17.0618, 16.2097)
  spline S338 degree 2 poles (17.0618, 16.2097) (17.0262, 16.2422) (16.916, 16.3329) (16.8365, 16.3767) knots 0 0 0 1 2 2 2
  spline S339 degree 2 poles (16.8365, 16.3767) (16.7604, 16.4188) (16.5805, 16.4723) (16.4638, 16.4723) knots 0 0 0 1 2 2 2
  spline S340 degree 2 poles (16.4638, 16.4723) (16.3357, 16.4723) (16.1072, 16.367) (16.0213, 16.2665) knots 0 0 0 1 2 2 2
  spline S341 degree 2 poles (16.0213, 16.2665) (15.937, 16.1644) (15.843, 15.8548) (15.843, 15.6619) knots 0 0 0 1 2 2 2
  spline S342 degree 2 poles (15.843, 15.6619) (15.843, 15.4561) (15.9419, 15.1595) (16.0278, 15.0574) knots 0 0 0 1 2 2 2
  spline S343 degree 2 poles (16.0278, 15.0574) (16.1121, 14.9585) (16.3373, 14.858) (16.4638, 14.858) knots 0 0 0 1 2 2 2
  spline S344 degree 2 poles (16.4638, 14.858) (16.5788, 14.858) (16.775, 14.9148) (16.8511, 14.9569) knots 0 0 0 1 2 2 2
  spline S345 degree 2 poles (16.8511, 14.9569) (16.9241, 14.999) (17.0326, 15.0866) (17.0634, 15.1174) knots 0 0 0 1 2 2 2
  line L496 (17.0634, 15.1174) -> (17.0829, 15.1174)
  line L497 (17.0829, 15.1174) -> (17.0829, 14.7997)
  spline S346 degree 2 poles (17.0829, 14.7997) (17.0164, 14.7689) (16.8997, 14.7122) (16.8171, 14.6862) knots 0 0 0 1 2 2 2
  spline S347 degree 2 poles (16.8171, 14.6862) (16.7296, 14.6571) (16.5805, 14.6279) (16.4605, 14.6279) knots 0 0 0 1 2 2 2
  line L498 (18.7831, 14.6636) -> (18.5173, 14.6636)
  line L499 (18.5173, 14.6636) -> (18.5173, 15.6425)
  line L500 (18.5173, 15.6425) -> (17.5967, 15.6425)
  line L501 (17.5967, 15.6425) -> (17.5967, 14.6636)
  line L502 (17.5967, 14.6636) -> (17.3309, 14.6636)
  line L503 (17.3309, 14.6636) -> (17.3309, 16.6636)
  line L504 (17.3309, 16.6636) -> (17.5967, 16.6636)
  line L505 (17.5967, 16.6636) -> (17.5967, 15.8791)
  line L506 (17.5967, 15.8791) -> (18.5173, 15.8791)
  line L507 (18.5173, 15.8791) -> (18.5173, 16.6636)
  line L508 (18.5173, 16.6636) -> (18.7831, 16.6636)
  line L509 (18.7831, 16.6636) -> (18.7831, 14.6636)
  line L510 (19.1882, 14.6636) -> (19.1882, 16.6636)
  line L511 (19.1882, 16.6636) -> (20.4395, 16.6636)
  line L512 (20.4395, 16.6636) -> (20.4395, 16.4269)
  line L513 (20.4395, 16.4269) -> (19.454, 16.4269)
  line L514 (19.454, 16.4269) -> (19.454, 15.8791)
  line L515 (19.454, 15.8791) -> (20.373, 15.8791)
  line L516 (20.373, 15.8791) -> (20.373, 15.6425)
  line L517 (20.373, 15.6425) -> (19.454, 15.6425)
  line L518 (19.454, 15.6425) -> (19.454, 14.9002)
  line L519 (19.454, 14.9002) -> (20.4395, 14.9002)
  line L520 (20.4395, 14.9002) -> (20.4395, 14.6636)
  line L521 (20.4395, 14.6636) -> (19.1882, 14.6636)
  spline S348 degree 2 poles (21.5124, 14.6279) (21.3179, 14.6279) (20.9889, 14.7592) (20.869, 14.8905) knots 0 0 0 1 2 2 2
  spline S349 degree 2 poles (20.869, 14.8905) (20.749, 15.0201) (20.6177, 15.4091) (20.6177, 15.6619) knots 0 0 0 1 2 2 2
  spline S350 degree 2 poles (20.6177, 15.6619) (20.6177, 15.9131) (20.7458, 16.2859) (20.8673, 16.4237) knots 0 0 0 1 2 2 2
  spline S351 degree 2 poles (20.8673, 16.4237) (20.9873, 16.5582) (21.3147, 16.6992) (21.5173, 16.6992) knots 0 0 0 1 2 2 2
  spline S352 degree 2 poles (21.5173, 16.6992) (21.6177, 16.6992) (21.7944, 16.67) (21.869, 16.6473) knots 0 0 0 1 2 2 2
  spline S353 degree 2 poles (21.869, 16.6473) (21.9338, 16.6263) (22.0683, 16.5663) (22.1348, 16.5307) knots 0 0 0 1 2 2 2
  line L522 (22.1348, 16.5307) -> (22.1348, 16.2097)
  line L523 (22.1348, 16.2097) -> (22.1137, 16.2097)
  spline S354 degree 2 poles (22.1137, 16.2097) (22.078, 16.2422) (21.9678, 16.3329) (21.8884, 16.3767) knots 0 0 0 1 2 2 2
  spline S355 degree 2 poles (21.8884, 16.3767) (21.8122, 16.4188) (21.6323, 16.4723) (21.5156, 16.4723) knots 0 0 0 1 2 2 2
  spline S356 degree 2 poles (21.5156, 16.4723) (21.3876, 16.4723) (21.1591, 16.367) (21.0732, 16.2665) knots 0 0 0 1 2 2 2
  spline S357 degree 2 poles (21.0732, 16.2665) (20.9889, 16.1644) (20.8949, 15.8548) (20.8949, 15.6619) knots 0 0 0 1 2 2 2
  spline S358 degree 2 poles (20.8949, 15.6619) (20.8949, 15.4561) (20.9938, 15.1595) (21.0797, 15.0574) knots 0 0 0 1 2 2 2
  spline S359 degree 2 poles (21.0797, 15.0574) (21.1639, 14.9585) (21.3892, 14.858) (21.5156, 14.858) knots 0 0 0 1 2 2 2
  spline S360 degree 2 poles (21.5156, 14.858) (21.6307, 14.858) (21.8268, 14.9148) (21.903, 14.9569) knots 0 0 0 1 2 2 2
  spline S361 degree 2 poles (21.903, 14.9569) (21.9759, 14.999) (22.0845, 15.0866) (22.1153, 15.1174) knots 0 0 0 1 2 2 2
  line L524 (22.1153, 15.1174) -> (22.1348, 15.1174)
  line L525 (22.1348, 15.1174) -> (22.1348, 14.7997)
  spline S362 degree 2 poles (22.1348, 14.7997) (22.0683, 14.7689) (21.9516, 14.7122) (21.869, 14.6862) knots 0 0 0 1 2 2 2
  spline S363 degree 2 poles (21.869, 14.6862) (21.7814, 14.6571) (21.6323, 14.6279) (21.5124, 14.6279) knots 0 0 0 1 2 2 2
  line L526 (23.8414, 14.6636) -> (23.4962, 14.6636)
  line L527 (23.4962, 14.6636) -> (22.7652, 15.5939)
  line L528 (22.7652, 15.5939) -> (22.6485, 15.4626)
  line L529 (22.6485, 15.4626) -> (22.6485, 14.6636)
  line L530 (22.6485, 14.6636) -> (22.3827, 14.6636)
  line L531 (22.3827, 14.6636) -> (22.3827, 16.6636)
  line L532 (22.3827, 16.6636) -> (22.6485, 16.6636)
  line L533 (22.6485, 16.6636) -> (22.6485, 15.7446)
  line L534 (22.6485, 15.7446) -> (23.4686, 16.6636)
  line L535 (23.4686, 16.6636) -> (23.7928, 16.6636)
  line L536 (23.7928, 16.6636) -> (22.9646, 15.7705)
  line L537 (22.9646, 15.7705) -> (23.8414, 14.6636)
  line L538 (18.6135, 4.7684) -> (17.7444, 4.7684)
  line L539 (17.7444, 4.7684) -> (17.7444, 6.2684)
  line L540 (17.7444, 6.2684) -> (17.9437, 6.2684)
  line L541 (17.9437, 6.2684) -> (17.9437, 4.9459)
  line L542 (17.9437, 4.9459) -> (18.6135, 4.9459)
  line L543 (18.6135, 4.9459) -> (18.6135, 4.7684)
  spline S364 degree 2 poles (19.8315, 6.097) (19.9166, 5.9973) (20.0114, 5.7056) (20.0114, 5.5184) knots 0 0 0 1 2 2 2
  spline S365 degree 2 poles (20.0114, 5.5184) (20.0114, 5.3361) (19.919, 5.0407) (19.8315, 4.941) knots 0 0 0 1 2 2 2
  spline S366 degree 2 poles (19.8315, 4.941) (19.7391, 4.8365) (19.4948, 4.7368) (19.3477, 4.7368) knots 0 0 0 1 2 2 2
  spline S367 degree 2 poles (19.3477, 4.7368) (19.1958, 4.7368) (18.9527, 4.8401) (18.8639, 4.941) knots 0 0 0 1 2 2 2
  spline S368 degree 2 poles (18.8639, 4.941) (18.7776, 5.0407) (18.6852, 5.3336) (18.6852, 5.5184) knots 0 0 0 1 2 2 2
  spline S369 degree 2 poles (18.6852, 5.5184) (18.6852, 5.7068) (18.7788, 5.9937) (18.8651, 6.097) knots 0 0 0 1 2 2 2
  spline S370 degree 2 poles (18.8651, 6.097) (18.9527, 6.1967) (19.197, 6.3) (19.3477, 6.3) knots 0 0 0 1 2 2 2
  spline S371 degree 2 poles (19.3477, 6.3) (19.5009, 6.3) (19.7464, 6.193) (19.8315, 6.097) knots 0 0 0 1 2 2 2
  spline S372 degree 2 poles (19.8035, 5.5184) (19.8035, 5.6667) (19.7391, 5.8964) (19.6808, 5.9718) knots 0 0 0 1 2 2 2
  spline S373 degree 2 poles (19.6808, 5.9718) (19.6212, 6.0496) (19.4535, 6.1274) (19.3489, 6.1274) knots 0 0 0 1 2 2 2
  spline S374 degree 2 poles (19.3489, 6.1274) (19.2407, 6.1274) (19.0779, 6.052) (19.0159, 5.9718) knots 0 0 0 1 2 2 2
  spline S375 degree 2 poles (19.0159, 5.9718) (18.9563, 5.8952) (18.8931, 5.6643) (18.8931, 5.5184) knots 0 0 0 1 2 2 2
  spline S376 degree 2 poles (18.8931, 5.5184) (18.8931, 5.223) (19.1411, 4.9094) (19.3489, 4.9094) knots 0 0 0 1 2 2 2
  spline S377 degree 2 poles (19.3489, 4.9094) (19.5568, 4.9094) (19.8035, 5.223) (19.8035, 5.5184) knots 0 0 0 1 2 2 2
  line L544 (20.0685, 4.7684) -> (20.5742, 6.2684)
  line L545 (20.5742, 6.2684) -> (20.8198, 6.2684)
  line L546 (20.8198, 6.2684) -> (21.3254, 4.7684)
  line L547 (21.3254, 4.7684) -> (21.1151, 4.7684)
  line L548 (21.1151, 4.7684) -> (20.979, 5.1878)
  line L549 (20.979, 5.1878) -> (20.4065, 5.1878)
  line L550 (20.4065, 5.1878) -> (20.2703, 4.7684)
  line L551 (20.2703, 4.7684) -> (20.0685, 4.7684)
  line L552 (20.9243, 5.3579) -> (20.6921, 6.0642)
  line L553 (20.6921, 6.0642) -> (20.4612, 5.3579)
  line L554 (20.4612, 5.3579) -> (20.9243, 5.3579)
  spline S378 degree 2 poles (22.6504, 5.5172) (22.6504, 5.3118) (22.4839, 4.9811) (22.3441, 4.8887) knots 0 0 0 1 2 2 2
  spline S379 degree 2 poles (22.3441, 4.8887) (22.2298, 4.817) (21.9952, 4.7684) (21.8129, 4.7684) knots 0 0 0 1 2 2 2
  line L555 (21.8129, 4.7684) -> (21.4676, 4.7684)
  line L556 (21.4676, 4.7684) -> (21.4676, 6.2684)
  line L557 (21.4676, 6.2684) -> (21.8092, 6.2684)
  spline S380 degree 2 poles (21.8092, 6.2684) (22.0207, 6.2684) (22.2614, 6.2052) (22.3465, 6.1493) knots 0 0 0 1 2 2 2
  spline S381 degree 2 poles (22.3465, 6.1493) (22.4911, 6.0532) (22.6504, 5.736) (22.6504, 5.5172) knots 0 0 0 1 2 2 2
  spline S382 degree 2 poles (22.4425, 5.5196) (22.4425, 5.6922) (22.3283, 5.9365) (22.2152, 6.0058) knots 0 0 0 1 2 2 2
  spline S383 degree 2 poles (22.2152, 6.0058) (22.135, 6.0532) (21.9539, 6.0958) (21.8189, 6.0958) knots 0 0 0 1 2 2 2
  line L558 (21.8189, 6.0958) -> (21.667, 6.0958)
  line L559 (21.667, 6.0958) -> (21.667, 4.941)
  line L560 (21.667, 4.941) -> (21.8189, 4.941)
  spline S384 degree 2 poles (21.8189, 4.941) (21.9514, 4.941) (22.152, 4.9835) (22.2334, 5.0407) knots 0 0 0 1 2 2 2
  spline S385 degree 2 poles (22.2334, 5.0407) (22.338, 5.1112) (22.4425, 5.3446) (22.4425, 5.5196) knots 0 0 0 1 2 2 2
  point P0 (0, 0)
  dimension "d411" = 5
  dimension "d412" = 8
  dimension "d420" = 4
  constraints: 6 collinear, 20 other
  measures "d411" distance from line of A0.centre L12
  measures "d412" distance from line of L8 A0.centre
  measures "d420" distance from line of A1.centre L21
extrude "Extrusión16" cut sketch "Boceto42" against normal blind 0.001 contours L40 L41 L42 L43 L44 L45 L46 L47 L48 L49 L50 L51 | L52 L53 L54 L55 L56 L57 L58 L59 L60 L61 | S0 S1 L62 L63 L64 L65 L66 S2 S3 | S8 S9 L70 L71 L72 S10 S11 S12 S13 L73 L74 L75 S14 S15 | L76 L77 L78 L79 L80 L81 L82 L83 | L84 L85 L86 L87 L88 L89 S16 L90 L91 L92 L93 | L94 L95 S17 S18 S19 S20 S21 S22 L96 L97 S23 S24 S25 S26 S27 L98 L99 | L100 L101 L102 L103 L104 L105 L106 | S28 S29 L107 L108 L109 L110 L111 S30 S31 | L115 L116 L117 L118 L119 L120 | S36 S37 L121 L122 L123 S38 S39 S40 S41 L124 L125 L126 S42 S43 | S44 S45 S46 S47 S48 S49 L127 L128 S50 S51 S52 S53 S54 S55 L129 L130 L131 L132 L133 S56 S57 | S58 S59 S60 S61 S62 S63 L134 L135 S64 S65 S66 S67 S68 S69 L136 L137 L138 L139 L140 S70 S71 | L141 L142 L143 L144 L145 L146 L147 L148 L149 L150 L151 L152 | S72 S73 L153 L154 L155 S74 S75 | L159 L160 L161 L162 L163 L164 L165 L166 | L167 L168 L169 L170 L171 L172 L173 L174 L175 L176 L177 L178 | S80 L179 L180 S81 S82 S83 S84 S85 S86 S87 S88 L181 L182 S89 S90 S91 S92 S93 S94 S95 | L183 L184 L185 L186 L187 L188 L189 L190 | L191 L192 L193 L194 L195 L196 L197 S96 S97 S98 L198 | L202 L203 L204 L205 L206 L207 L208 L209 L210 L211 L212 L213 | S103 L214 L215 S104 S105 S106 S107 S108 S109 S110 S111 L216 L217 S112 S113 S114 S115 S116 S117 S118 | S119 S120 L218 L219 L220 S121 S122 S123 S124 L221 L222 L223 S125 S126 | L224 L225 L226 L227 L228 L229 | L230 L231 L232 L233 L234 L235 L236 L237 | S127 L238 L239 S128 S129 S130 S131 S132 S133 S134 S135 L240 L241 S136 S137 S138 S139 S140 S141 S142 | S143 S144 L242 L243 L244 L245 L246 S145 S146 | L250 L251 L252 L253 L254 L255 L256 L257 | S151 L261 L262 S152 S153 S154 S155 S156 S157 S158 S159 L263 L264 S160 S161 S162 S163 S164 S165 S166 | S167 L265 L266 S168 S169 S170 S171 S172 S173 S174 S175 L267 L268 S176 S177 S178 S179 S180 S181 S182 | L269 L270 L271 L272 L273 L274 L275 L276 L277 L278 | L279 L280 L281 L282 L283 L284 L285 L286 | L290 L291 L292 L293 L294 L295 L296 L297 L298 L299 L300 L301 | L302 L303 L304 L305 L306 L307 | S183 S184 S185 L308 S186 S187 S188 S189 L309 S190 S191 | L310 S202 S203 S204 S205 L311 L312 L313 L314 S206 S207 S208 S209 L315 L316 L317 | L318 L319 L320 L321 L322 L323 L324 L325 L326 L327 L328 L329 | L330 L331 L332 L333 | L334 L335 L336 L337 L338 L339 S210 L340 L341 L342 L343 | S211 S212 S213 S214 | S223 S224 S225 S226 | S227 S228 S229 S230 | L344 L345 L346 L347 | S239 S240 L348 L349 L350 L351 L352 S241 S242 | S247 S248 L356 L357 L358 S249 S250 S251 S252 L359 L360 L361 S253 S254 | S255 L362 L363 S256 S257 S258 S259 S260 S261 S262 S263 L364 L365 S264 S265 S266 S267 S268 S269 S270 | L366 L367 L368 L369 L370 L371 L372 L373 L374 L375 L376 L377 | L378 L379 L380 L381 L382 L383 | S271 S272 S273 S274 S275 S276 S277 S278 | L384 L385 L386 L387 L388 L389 L390 L391 | S285 S286 L395 L396 L397 S287 S288 | S293 S294 S295 S296 S297 S298 L401 L402 S299 S300 S301 S302 S303 S304 S305 S306 L403 L404 S307 S308 | L405 L406 L407 L408 L409 L410 L411 L412 L413 L414 L415 L416 | L417 L418 L419 L420 L421 L422 L423 L424 L425 L426 L427 L428 | S309 S310 S311 S312 S313 S314 L429 L430 S315 S316 S317 S318 S319 S320 S321 S322 L431 L432 S323 S324 | L433 L434 L435 L436 L437 L438 L439 L440 L441 L442 L443 L444 | L445 L446 L447 L448 L449 L450 L451 S325 S326 S327 L452 | L456 L457 L458 L459 L460 L461 L462 L463 L464 L465 L466 L467 | L468 L474 L473 | L473 L474 L475 L476 L477 L478 L479 L480 L481 | L468 L469 L470 L471 L472 L473 L474 | L485 L486 L487 L488 L489 L490 L491 L492 L493 | S332 S333 S334 S335 S336 S337 L494 L495 S338 S339 S340 S341 S342 S343 S344 S345 L496 L497 S346 S347 | L498 L499 L500 L501 L502 L503 L504 L505 L506 L507 L508 L509 | L510 L511 L512 L513 L514 L515 L516 L517 L518 L519 L520 L521 | S348 S349 S350 S351 S352 S353 L522 L523 S354 S355 S356 S357 S358 S359 S360 S361 L524 L525 S362 S363 | L526 L527 L528 L529 L530 L531 L532 L533 L534 L535 L536 L537 | L538 L539 L540 L541 L542 L543 | S364 S365 S366 S367 S368 S369 S370 S371 | L544 L545 L546 L547 L548 L549 L550 L551 | S378 S379 L555 L556 L557 S380 S381
sketch "Boceto44" plane through (0, 0, 2) normal (0, 0, 1) x (1, 0, 0)
  line L0 (34, 35) -> (-34, 35) projected
  line L1 (25, 20) -> (-25, 20) projected
  line L2 (-2.9167, 30) -> (2.9167, 30) construction
  line L3 (2.9167, 30) -> (2.9167, 24) construction
  line L4 (2.9167, 24) -> (-2.9167, 24) construction
  line L5 (-2.9167, 24) -> (-2.9167, 30) construction
  line L6 (-2.9167, 26.5) -> (-1.6167, 26.5)
  line L7 (-1.6167, 26.5) -> (-1.6167, 25.5)
  line L8 (-1.6167, 25.5) -> (-2.9167, 25.5)
  line L9 (-2.9167, 25.5) -> (-2.9167, 26.5)
  line L10 (-1.5167, 25.5) -> (-0.5167, 25.5)
  line L11 (-0.5167, 25.5) -> (-0.5167, 24)
  line L12 (-0.5167, 24) -> (-1.5167, 24)
  line L13 (-1.5167, 24) -> (-1.5167, 25.5)
  line L14 (-0.4167, 25.5) -> (1.6833, 25.5)
  line L15 (1.6833, 25.5) -> (2.9167, 26.7333)
  line L16 (2.9167, 26.7333) -> (2.9167, 28.7667)
  line L17 (2.9167, 28.7667) -> (1.6833, 30)
  line L18 (1.6833, 30) -> (-0.2833, 30)
  line L19 (-1.5167, 28.7667) -> (-0.2833, 30)
  line L20 (-1.5167, 28.7667) -> (-1.5167, 26.5)
  line L21 (-0.5167, 26.5) -> (-1.5167, 26.5)
  line L22 (-0.4167, 26.5) -> (1.2691, 26.5)
  line L23 (1.2691, 26.5) -> (1.9167, 27.1475)
  line L24 (1.9167, 27.1475) -> (1.9167, 28.3525)
  line L25 (1.9167, 28.3525) -> (1.2691, 29)
  line L26 (1.2691, 29) -> (0.1309, 29)
  line L27 (0.1309, 29) -> (-0.5167, 28.3525)
  line L28 (-0.5167, 28.3525) -> (-0.5167, 26.5)
  line L29 (-0.4167, 26.5) -> (-0.4167, 25.5)
  point P0 (0, 0)
  point P1 (0, 35)
  point P2 (0, 35)
  point P3 (0, 30)
  dimension "d449" = 5
  dimension "d450" = 6
  dimension "d451" = 1
  dimension "d452" = 3.5
  dimension "d453" = 1.3
  dimension "d454" = 1
  dimension "d455" = 0.1
  dimension "d457" = 45
  dimension "d461" = 0.1
  dimension "d463" = 1
  dimension "d464" = 1
  dimension "d465" = 1
  dimension "d466" = 1
  dimension "d467" = 1
  dimension "d468" = 4.6
  constraints: 48 end point, 8 perpendicular, 7 parallel, 6 collinear, 6 point on line, 4 horizontal, 3 midpoint, 3 vertical, 1 vertical alignment, 2 other
  measures "d449" distance between parallel lines of L0 L2
  measures "d450" distance of L2.end L3.end
  measures "d451" distance between parallel lines of L8 L6
  measures "d452" distance between parallel lines of L2 L6
  measures "d453" distance of L7.end L8.end
  measures "d454" distance between parallel lines of L13 L11
  measures "d455" distance between parallel lines of L7 L13
  measures "d457" angle of L23 L22
  measures "d461" distance between parallel lines of L29 L11
  measures "d463" distance between parallel lines of L15 L23
  measures "d464" distance between parallel lines of L19 L27
  measures "d465" distance between parallel lines of L2 L26
  measures "d466" distance between parallel lines of L16 L24
  measures "d467" distance between parallel lines of L17 L25
  measures "d468" distance from line of L5 L14.end
extrude "Extrusión17" add sketch "Boceto44" along normal blind 0.001